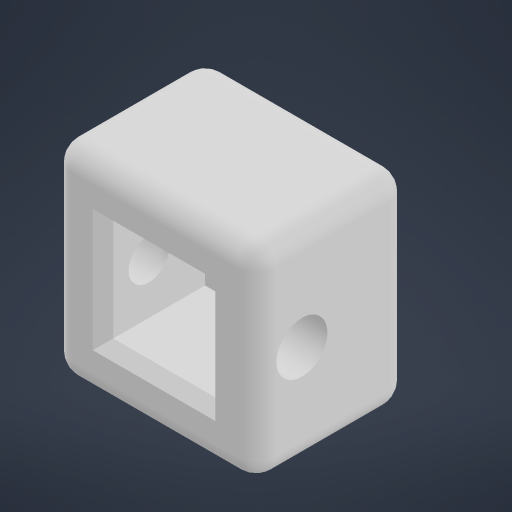
# Autodesk Inventor part: Clamp_Adapter_V1
Saved by Autodesk Inventor 2024 (Build 280153000, 153)
## iProperties
Created: 2023-07-01
Part Number: Clamp_Adapter_V1
Material: Generic
Document SubType Name: Modeling
Designer: User
Density: 1 g/cm^3
Appearance: Default
Author: User
Autodesk Inventor part; units mm, degrees
ref_plane "YZ Plane" through (0, 0, 0) normal (1, 0, 0) x (0, 1, 0)
ref_plane "XZ Plane" through (0, 0, 0) normal (0, 1, 0) x (-1, 0, 0)
ref_plane "XY Plane" through (0, 0, 0) normal (0, 0, 1) x (1, 0, 0)
sketch "Sketch14" plane through (0, 0, 0) normal (0, 0, 1) x (1, 0, 0)
  line L0 (0, 0) -> (-20, 0)
  line L1 (-20, 0) -> (-20, 20)
  line L2 (-20, 20) -> (0, 20)
  line L3 (0, 20) -> (0, 0)
  line L4 (-5, 5) -> (-10, 5)
  line L5 (-10, 5) -> (-10, 10)
  line L6 (-10, 10) -> (-5, 10)
  line L7 (-5, 10) -> (-5, 5)
  dimension "d71" = 20
  dimension "d72" = 20
  dimension "d73" = 5
  dimension "d74" = 5
  constraints: 16 end point, 4 parallel, 2 horizontal, 2 perpendicular
  measures "d71" distance of L1.end L2.end
  measures "d72" distance of L0.end L1.end
  measures "d73" distance of L5.end L6.end
  measures "d74" distance of L4.end L5.end
extrude "Extrusion9" add sketch "Sketch14" along normal blind 15 contours L0 L1 L2 L3 | L4 L5 L6 L7
fillet "Fillet1" radius 2 12 edges at (-20, 20, 7.5) (-20, 10, 0) (-20, 0, 7.5) (-20, 10, 15) (0, 10, 15) (-10, 20, 15) (0, 20, 7.5) (-10, 20, 0) (-10, 0, 15) (0, 10, 0) (0, 0, 7.5) (-10, 0, 0)
sketch "Sketch19" plane through (0, 0, 0) normal (0, 0, -1) x (-1, 0, 0)
  line L0 (17, 3) -> (12.5, 3)
  line L1 (12.5, 3) -> (12.5, 7.5)
  line L2 (12.5, 7.5) -> (17, 7.5)
  line L3 (17, 7.5) -> (17, 3)
  point P0 (0, 0)
  point P1 (20, 20)
  dimension "d164" = 4.5
  dimension "d165" = 4.5
  constraints: 8 end point, 2 parallel, 1 horizontal, 1 perpendicular
  measures "d164" distance of L1.end L2.end
  measures "d165" distance of L0.end L1.end
extrude "Extrusion15" add sketch "Sketch19" along normal blind 5
chamfer "Chamfer12" distance 1 angle 45 4 edges at (-17, 5.25, -5) (-14.75, 7.5, -5) (-12.5, 5.25, -5) (-14.75, 3, -5)
sketch "Sketch24" plane through (0, 0, 15) normal (0, 0, 1) x (1, 0, 0)
  line L0 (-15, 15) -> (-5, 15)
  line L1 (-5, 15) -> (-5, 5)
  line L2 (-5, 5) -> (-15, 5)
  line L3 (-15, 5) -> (-15, 15)
  point P0 (0, 0)
  dimension "d176" = 10
  dimension "d177" = 10
  constraints: 8 end point, 2 parallel, 1 horizontal, 1 perpendicular
  measures "d176" distance of L1.end L2.end
  measures "d177" distance of L0.end L1.end
extrude "Extrusion16" cut sketch "Sketch24" against normal blind 10
chamfer "Chamfer13" distance 1 angle 45 4 edges at (-10, 5, 15) (-5, 10, 15) (-10, 15, 15) (-15, 10, 15)
sketch "Sketch28" plane through (-20, 2, 2) normal (-1, 0, 0) x (0, 0, 1)
  point P0 (-2, -2)
  point P1 (8.5, 8)
hole "Hole15" at (-20, 10, 10.5) direction (1, 0, 0) diameter 4 depth 6 counterbore diameter 5 counterbore depth 4.5
sketch "Sketch29" plane through (0, 2, 13) normal (1, 0, 0) x (0, 0, -1)
  circle A0 centre (2.5, 8) radius 2 projected
  point P0 (13, -2)
  constraints: 1 coincident
hole "Hole16" at (0, 10, 10.5) direction (-1, 0, 0) diameter 4 depth 6 counterbore diameter 5 counterbore depth 4.5
body "Solid4"
